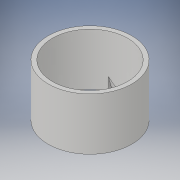
# Autodesk Inventor part: Whistle Splitter 40mmR
Saved by Autodesk Inventor 2019 (Build 230136000, 136)
## iProperties
Created: 2020-04-08
Part Number: Whistle Splitter 40mmR
Material: Generic
Document SubType Name: Modeling
Designer: Kepler
Density: 1 g/cm^3
Appearance: Default
Author: Kepler
Autodesk Inventor part; units mm, degrees
ref_plane "YZ Plane" through (0, 0, 0) normal (1, 0, 0) x (0, 1, 0)
ref_plane "XZ Plane" through (0, 0, 0) normal (0, 1, 0) x (-1, 0, 0)
ref_plane "XY Plane" through (0, 0, 0) normal (0, 0, 1) x (1, 0, 0)
sketch "Sketch1" plane through (0, 0, 0) normal (0, 1, 0) x (-1, 0, 0)
  circle A0 centre (0, 0) radius 40
  circle A1 centre (0, 0) radius 36
  dimension "d1" = 72
  dimension "d8" = 80
  constraints: 2 centre point, 2 coincident
  measures "d1" diameter of A1
  measures "d8" diameter of A0
extrude "Extrusion1" add sketch "Sketch1" along normal blind 50
sketch "Sketch2" plane through (0, 0, 0) normal (1, 0, 0) x (0, 1, 0)
  line L0 (0, 40) -> (0, -40) projected
  line L1 (0, -36) -> (19.3804, -30.807)
  line L2 (0, -36) -> (20.8201, -41.5787)
  line L3 (19.3804, -30.807) -> (-2.465, -30.807)
  line L4 (-2.465, -30.807) -> (-2.465, -42.37)
  line L5 (-2.465, -42.37) -> (20.8201, -42.37)
  line L6 (20.8201, -42.37) -> (20.8201, -41.5787)
  line L7 (0, -36) -> (50, -36) projected
  point P0 (0, 0)
  dimension "d6" = 15
  dimension "d7" = 15
  constraints: 12 end point, 3 perpendicular, 1 horizontal
  measures "d6" angle of L2 L7
  measures "d7" angle of L7 L1
extrude "Extrusion2" cut sketch "Sketch2" along normal mid plane 30
body "Solid1"
